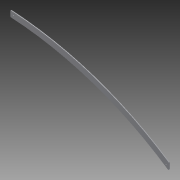
# Autodesk Inventor part: Ramp
Saved by Autodesk Inventor 2014 (Build 180170000, 170)
## iProperties
Created: 2014-01-20
Part Number: Ramp
Material: Aluminum 6061
Document SubType Name: Modeling
Designer: Andrew Toennies
Mass: 159.972 g
Surface Area: 419.88 cm^2
Volume: 59.0303 cm^3
Density: 2.71 g/cm^3
Appearance: Aluminum - Flat
Author: Andrew Toennies
Autodesk Inventor part; units mm, degrees
ref_plane "YZ Plane" through (0, 0, 0) normal (1, 0, 0) x (0, 1, 0)
ref_plane "XZ Plane" through (0, 0, 0) normal (0, 1, 0) x (-1, 0, 0)
ref_plane "XY Plane" through (0, 0, 0) normal (0, 0, 1) x (1, 0, 0)
sketch "Sketch1" plane through (0, 0, 0) normal (0, 0, 1) x (1, 0, 0)
  line L0 (342.9, 44.45) -> (342.9, 717.1861) construction
  line L1 (-606.2082, 101.6) -> (1077.8216, 101.6) construction
  line L2 (-65.7713, 44.45) -> (606.7605, 44.45) construction
  line L3 (-222.4708, -127) -> (709.547, -127) construction
  arc A0 (684.6761, -149.4566) -> (3.1862, 101.5935) centre (-0.5715, -959.104) ccw
  arc A1 (680.5362, -179.3945) -> (3.1635, 76.1934) centre (-0.5715, -959.104) ccw
  line L4 (0, 98.4185) -> (0, 79.3684)
  arc A2 (3.1862, 101.5935) -> (0, 98.4185) centre (3.175, 98.4185) ccw
  arc A3 (0, 79.3684) -> (3.1635, 76.1934) centre (3.175, 79.3684) ccw
  line L5 (685.8, 390.8172) -> (685.8, -177.0033) construction
  line L6 (657.225, 88.3294) -> (657.225, -181.9974) construction
  line L7 (685.8, -177.0033) -> (685.8, -151.8801)
  arc A4 (685.8, -151.8801) -> (684.6761, -149.4566) centre (682.625, -151.8801) ccw
  arc A5 (680.5362, -179.3945) -> (685.8, -177.0033) centre (682.625, -177.0033) ccw
  point P0 (0, 0)
  point P1 (0, 101.6)
  point P2 (850.5097, -369.5996)
  point P3 (0, 76.2)
  point P4 (685.8, -184.0241)
  point P5 (657.225, -127)
  point P6 (685.8, -150.4091)
  dimension "d2" = 342.9
  dimension "d3" = 101.6
  dimension "d4" = 44.45
  dimension "d6" = 127
  dimension "d7" = 25.4
  dimension "d9" = 3.175
  dimension "d20" = 685.8
  dimension "d21" = 657.225
  dimension "d22" = 3.175
  constraints: 20 point on circle, 16 end point, 10 point on line, 8 tangent, 6 centre point, 3 vertical, 2 equal radius, 2 horizontal, 2 parallel, 1 perpendicular
  measures "d2" distance from line of point (0, 0) L0
  measures "d3" distance from line of point (0, 0) L1
  measures "d4" distance from line of point (0, 0) L2
  measures "d6" distance from line of point (0, 0) L3
  measures "d7" radial gap between concentric circles of A0 A1
  measures "d9" radius of A2
  measures "d20" distance from line of point (0, 0) L5
  measures "d21" distance from line of point (0, 0) L6
  measures "d22" radius of A4
extrude "Extrusion1" add sketch "Sketch1" along normal blind 3.175
sketch "Sketch2" plane through (0, 0, 0) normal (0, 0, -1) x (-1, 0, 0)
  line L0 (0, 79.3684) -> (0, 98.4185) projected
  circle A0 centre (-12.7, 88.9) radius 2.0701
  circle A1 centre (-673.1, -165.1) radius 2.0701
  point P0 (0, 0)
  dimension "d12" = 4.1402
  dimension "d13" = 12.7
  dimension "d14" = 88.9
  dimension "d15" = 4.1402
  dimension "d17" = 165.1
  dimension "d23" = 673.1
  constraints: 2 centre point
  measures "d12" diameter of A0
  measures "d13" distance from line of L0 A0.centre
  measures "d14" vertical distance of point (0, 0) A0.centre
  measures "d15" diameter of A1
  measures "d17" vertical distance of point (0, 0) A1.centre
  measures "d23" horizontal distance of point (0, 0) A1.centre
extrude "Extrusion2" cut sketch "Sketch2" against normal blind 25.4
sketch "Sketch3" plane through (0, 0, 0) normal (0, 0, -1) x (-1, 0, 0)
  arc A0 (-3.1862, 101.5935) -> (-684.6761, -149.4566) centre (0.5715, -959.104) ccw projected
  arc A1 (-3.1635, 76.1934) -> (-680.5362, -179.3945) centre (0.5715, -959.104) ccw projected
  line L0 (0, 79.3684) -> (0, 98.4185) projected
  circle A2 centre (-36.0033, 88.2616) radius 6.35
  line L1 (-36.0033, 88.2616) -> (0.5715, -959.104) construction
  line L2 (0.5715, -959.104) -> (0.5715, -266.0692) construction
  line L3 (0.5715, -959.104) -> (-683.9382, -148.8325) construction
  circle A3 centre (-53.34, 87.5124) radius 6.35
  circle A4 centre (-70.662, 86.4763) radius 6.35
  circle A5 centre (-87.9644, 85.1535) radius 6.35
  circle A6 centre (-105.2426, 83.5444) radius 6.35
  circle A7 centre (-122.4917, 81.6495) radius 6.35
  circle A8 centre (-139.7071, 79.4692) radius 6.35
  circle A9 centre (-156.8841, 77.0042) radius 6.35
  circle A10 centre (-174.0178, 74.2551) radius 6.35
  circle A11 centre (-191.1037, 71.2226) radius 6.35
  circle A12 centre (-208.1371, 67.9077) radius 6.35
  circle A13 centre (-225.1132, 64.3113) radius 6.35
  circle A14 centre (-242.0275, 60.4342) radius 6.35
  circle A15 centre (-258.8752, 56.2776) radius 6.35
  circle A16 centre (-275.6518, 51.8426) radius 6.35
  circle A17 centre (-292.3527, 47.1305) radius 6.35
  circle A18 centre (-308.9733, 42.1424) radius 6.35
  circle A19 centre (-325.509, 36.8799) radius 6.35
  circle A20 centre (-341.9553, 31.3443) radius 6.35
  circle A21 centre (-358.3077, 25.5371) radius 6.35
  circle A22 centre (-374.5617, 19.46) radius 6.35
  circle A23 centre (-390.7128, 13.1146) radius 6.35
  circle A24 centre (-406.7567, 6.5026) radius 6.35
  circle A25 centre (-422.6889, -0.3741) radius 6.35
  circle A26 centre (-438.505, -7.5136) radius 6.35
  circle A27 centre (-454.2008, -14.9141) radius 6.35
  circle A28 centre (-469.7718, -22.5734) radius 6.35
  circle A29 centre (-485.214, -30.4895) radius 6.35
  circle A30 centre (-500.5229, -38.6602) radius 6.35
  circle A31 centre (-515.6944, -47.0832) radius 6.35
  circle A32 centre (-530.7245, -55.7563) radius 6.35
  circle A33 centre (-545.6088, -64.6771) radius 6.35
  circle A34 centre (-560.3434, -73.8431) radius 6.35
  circle A35 centre (-574.9242, -83.2518) radius 6.35
  circle A36 centre (-589.3472, -92.9006) radius 6.35
  circle A37 centre (-603.6085, -102.787) radius 6.35
  circle A38 centre (-617.7042, -112.908) radius 6.35
  circle A39 centre (-631.6303, -123.2611) radius 6.35
  circle A40 centre (-645.3831, -133.8434) radius 6.35
  circle A41 centre (-658.9588, -144.6519) radius 6.35
  point P0 (0, 0)
  dimension "d24" = 12.7
  dimension "d25" = 1048.004
  dimension "d26" = 2
  dimension "d27" = 40.191
  dimension "d30" = 37
  constraints: 40 centre point, 6 end point, 1 parallel, 1 point on circle, 79 other
  measures "d24" diameter of A2
  measures "d25" distance of L1.start L1.end
  measures "d26" angle of L1 L2
  measures "d27" angle of L3 L2
extrude "Extrusion3" cut sketch "Sketch3" against normal blind 25.4
body "Solid1"
